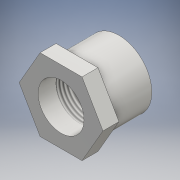
# Autodesk Inventor part: PVCConnectorFemale3_4inch
Saved by Autodesk Inventor 2016 (Build 200138000, 138)
## iProperties
Created: 2015-11-15
Part Number: PVCConnectorFemale3_4inch
Material: PVC-Piping
Document SubType Name: Modeling
Designer: Artur
Density: 1.4 g/cm^3
Appearance: Smooth - White
Mass: 26.4063 g
Surface Area: 66.4215 cm^2
Volume: 18.8616 cm^3
Author: Artur
Autodesk Inventor part; units mm, degrees
ref_plane "YZ Plane" through (0, 0, 0) normal (1, 0, 0) x (0, 1, 0)
ref_plane "XZ Plane" through (0, 0, 0) normal (0, 1, 0) x (-1, 0, 0)
ref_plane "XY Plane" through (0, 0, 0) normal (0, 0, 1) x (1, 0, 0)
sketch "Sketch1" plane through (0, 0, 0) normal (0, 1, 0) x (-1, 0, 0)
  circle A0 centre (0, 0) radius 16.5
  circle A1 centre (0, 0) radius 11.5
  dimension "d0" = 33
  dimension "d1" = 23
  constraints: 2 centre point, 2 coincident
  measures "d0" diameter of A0
  measures "d1" diameter of A1
extrude "tappedEnd" add sketch "Sketch1" along normal blind 21
thread "Thread1" size "3/4" designation "3/4 - 14 NPT" standard "NPT for PVC Pipe and Fitting" length 20.155
sketch "Sketch2" plane through (0, 0, 0) normal (0, -1, 0) x (1, 0, 0)
  circle A0 centre (0, 0) radius 21 construction
  line L0 (-10.5, 18.1865) -> (10.5, 18.1865)
  line L1 (10.5, 18.1865) -> (21, 0)
  line L2 (21, 0) -> (10.5, -18.1865)
  line L3 (10.5, -18.1865) -> (-10.5, -18.1865)
  line L4 (-10.5, -18.1865) -> (-21, 0)
  line L5 (-21, 0) -> (-10.5, 18.1865)
  circle A1 centre (0, 0) radius 11.5 projected
  dimension "d6" = 42
  constraints: 12 end point, 6 point on circle, 4 equal length, 1 centre point, 1 coincident, 1 horizontal, 1 parallel
  measures "d6" diameter of A0
extrude "hexBit" add sketch "Sketch2" along normal blind 8
sketch "Sketch3" plane through (0, -8, 0) normal (0, -1, 0) x (1, 0, 0)
  circle A0 centre (0, 0) radius 11.5 projected
  circle A1 centre (0, 0) radius 16.5
  dimension "d9" = 33
  constraints: 1 centre point, 1 coincident
  measures "d9" diameter of A1
extrude "Extrusion3" [suppressed]
body "Solid1"
